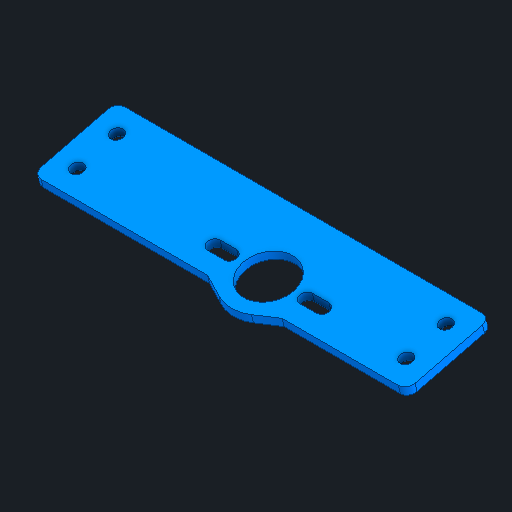
# Autodesk Inventor part: motor_mount_plate
Saved by Autodesk Inventor 2023 (Build 270158030, 158C)
## iProperties
Created: 2022-03-30
Part Number: motor_mount_plate
Material: Generic
Document SubType Name: Modeling
Designer: kardo
Density: 1 g/cm^3
Appearance: Blue Plastic
Author: kardo
Autodesk Inventor part; units mm, degrees
ref_plane "YZ Plane" through (0, 0, 0) normal (1, 0, 0) x (0, 1, 0)
ref_plane "XZ Plane" through (0, 0, 0) normal (0, 1, 0) x (-1, 0, 0)
ref_plane "XY Plane" through (0, 0, 0) normal (0, 0, 1) x (1, 0, 0)
derived "stencil_frame.ipt"
sketch "sk_cowl_joint_locations" plane through (54.6, 0, 0) normal (1, 0, 0) x (0, 1, 0)
  line L0 (-363, 18.496) -> (-275.8801, 20.463) construction
  arc A0 (-275.8801, 20.463) -> (-254.1001, 21.0191) centre (-359.1231, 3707.4463) ccw construction
  line L1 (-254.1001, 21.0191) -> (9.48, 28.5282) construction
  arc A1 (30.81, 28.832) -> (9.48, 28.5282) centre (30.81, -720.1791) ccw construction
  line L2 (30.81, 28.832) -> (94.8, 28.832) construction
  line L3 (94.8, 30.032) -> (30.81, 30.032) construction
  arc A2 (30.81, 30.032) -> (9.4458, 29.7277) centre (30.81, -720.1791) ccw construction
  line L4 (9.4458, 29.7277) -> (-254.1343, 22.2186) construction
  arc A3 (-275.9072, 21.6626) -> (-254.1343, 22.2186) centre (-359.1231, 3707.4463) ccw construction
  line L5 (-275.9072, 21.6626) -> (-363, 19.6963) construction
  line L6 (-242.0001, 4666.1952) -> (-242.0001, -2045.0469) construction
  line L7 (-120.9999, 4666.1952) -> (-120.9999, -2045.0469) construction
  line L8 (-363, 4666.1952) -> (-363, -2045.0469) construction
  line L9 (0, 4666.1952) -> (0, -2045.0469) construction
  line L10 (-242.0001, 45.0688) -> (-242.0001, 22.5643) construction
  line L11 (-120.9999, 49.9661) -> (-120.9999, 26.0115) construction
  line L12 (-363, 19.6963) -> (-363, 19.6963)
  line L13 (-363, 19.6963) -> (-363, 36.9211) construction
  line L14 (-1246.9714, 4491.7596) -> (383.4376, -2047.4538) construction
  line L15 (-362.7741, 36.9211) -> (-363, 39.712) construction
  line L16 (0, 51.6) -> (0, 29.4586) construction
  line L17 (-142.5135, 45.4866) -> (-137.5404, 25.5402) construction
  line L18 (-134.9025, 31.4945) -> (-138.7836, 30.5268) construction
  line L19 (-137.3891, 41.4677) -> (-141.2702, 40.5) construction
  line L20 (-142.5135, 45.4866) -> (-138.6324, 46.4543) construction
  line L21 (-137.5404, 25.5402) -> (-133.6592, 26.5079) construction
  line L22 (-138.6324, 46.4543) -> (-138.8117, 52.2515) construction
  spline S0 degree 2 poles (-363, 39.712) (-181.6483, 54.394) (0, 54.4) knots 0 0 0 1 1 1
  spline S1 degree 3 poles (0, 54.4) (31.284, 54.4) (68.256, 47.9917) (94.8, 37.536) knots 1 1 1 1 2 2 2 2
  spline S2 degree 3 poles (93.7738, 34.9308) (89.4268, 36.6431) (81.2968, 39.4556) (71.234, 42.2519) (63.4432, 44.1558) (58.1419, 45.3261) (51.4169, 46.6598) (45.9725, 47.6212) (39.1225, 48.6857) (33.6211, 49.4253) (26.7536, 50.2046) (21.2812, 50.7098) (14.5037, 51.1886) (7.8073, 51.5121) (2.5751, 51.6) (0, 51.6) knots 1 1 1 1 1.166667 1.291667 1.333333 1.416667 1.458333 1.541667 1.583333 1.666667 1.708333 1.791667 1.833333 1.916667 2 2 2 2
  spline S3 degree 3 poles (0, 51.6) (-20.1706, 51.5993) (-55.4643, 51.3605) (-95.7903, 50.6123) (-126.0307, 49.8474) (-146.1889, 49.2356) (-171.3841, 48.3435) (-191.5382, 47.528) (-216.7283, 46.3813) (-236.8783, 45.3621) (-262.0632, 43.9608) (-282.2091, 42.7379) (-307.3889, 41.082) (-332.5661, 39.2987) (-352.7052, 37.7363) (-362.7741, 36.9211) knots 0 0 0 0 0.166667 0.291667 0.333333 0.416667 0.458333 0.541667 0.583333 0.666666 0.708333 0.791666 0.833333 0.916666 1 1 1 1
  point P0 (0, 0)
  point P1 (-363, 28.3087)
  point P2 (-242.0001, 33.8165)
  point P3 (-120.9999, 37.9888)
  point P4 (0, 40.5293)
  point P5 (0, 40.5293)
ref_plane "plane_motor_mount" through (0, -127.05, 0) normal (0, 0.9702957, 0.2419219) x (-1, 0, 0)
ref_plane "plane_symmetry" through (0, 0, 0) normal (1, 0, 0) x (0, 1, 0)
sketch "sk_drivetrain_profile" plane through (6, 0, 0) normal (1, 0, 0) x (0, 1, 0)
  line L0 (-547.3485, 0) -> (393.091, 0) construction
  line L1 (-363, 4666.1952) -> (-363, -2045.0469) construction
  line L2 (0, 4666.1952) -> (0, -2045.0469) construction
  line L3 (-140.6277, 54.4571) -> (-133.8539, 27.2888)
  line L4 (-388, 0) -> (-343.0839, 2.7472)
  line L5 (-137.2408, 40.8729) -> (-226.9463, 18.5069)
  line L6 (-320.2745, 4.1423) -> (-272.9504, 7.0367) construction
  line L7 (-272.9504, 7.0367) -> (-226.9463, 18.5069) construction
  line L8 (-133.8539, 27.2888) -> (-133.8539, 22.2888) construction
  line L9 (-343.0839, 2.7472) -> (-320.2745, 4.1423)
  line L10 (-1246.9714, 4491.7596) -> (383.4376, -2047.4538) construction
  line L11 (-227.5223, 20.8174) -> (-137.8168, 43.1835) construction
  line L12 (-136.6647, 38.5624) -> (-226.3702, 16.1963) construction
  line L13 (-227.5223, 20.8174) -> (-226.3702, 16.1963) construction
  spline S0 degree 2 poles (-320.2745, 4.1423) (-272.9504, 7.0367) (-226.9463, 18.5069) knots 1 1 1 2 2 2
  line L14 (0, 21.4767) -> (-254.1001, 20.7404) construction
  line L15 (-55.6943, 22.5153) -> (-309.842, 21.7788) construction
  point P0 (0, 0)
  point P1 (-217.5636, 20.8462)
  point P2 (-207.6048, 20.8751)
  point P3 (-202.7352, 22.0892)
derived "parameters_frame.ipt"
sketch "sk_base" plane through (0, -127.05, 0) normal (0, 0.9702957, 0.2419219) x (-1, 0, 0)
  line L0 (0, -1635.5292) -> (0, 4543.1118) projected
  line L1 (-44.6, 47.8764) -> (-44.6, 27.3194)
  line L2 (-44.6, 27.3194) -> (0, 27.3194)
  line L3 (-44.6, 47.8764) -> (0, 47.8764)
  point P0 (0, -30.7362)
  point P1 (-54.6, 47.8764)
  point P2 (-54.6, 27.3194)
  dimension "d1" = 10
  constraints: 6 end point, 4 point on line, 2 perpendicular, 1 parallel
  measures "d1" distance from line of point (-54.6, 47.876) L1
extrude "base" add sketch "sk_base" against normal blind 2
sketch "sk_drill_joint" plane through (0, -127.05, 0) normal (0, 0.9702957, 0.2419219) x (-1, 0, 0)
  line L0 (-44.6, 47.8764) -> (-44.6, 27.3194) construction
  line L1 (-44.6, 47.8764) -> (0, 47.8764) construction
  line L2 (-44.6, 27.3194) -> (0, 27.3194) construction
  circle A0 centre (-39.2, 32.7194) radius 1.5
  circle A1 centre (-39.2, 42.4764) radius 1.5
  line L3 (-39.2, 42.4764) -> (-39.2, 47.8764) construction
  line L4 (-39.2, 42.4764) -> (-39.2, 32.7194) construction
  line L5 (-39.2, 32.7194) -> (-39.2, 27.3194) construction
  line L6 (-39.2, 42.4764) -> (-44.6, 42.4764) construction
  line L7 (-39.2, 32.7194) -> (-44.6, 32.7194) construction
  point P0 (0, -30.7362)
  dimension "d3" = 3
  dimension "d4" = 5.4
  constraints: 10 end point, 4 perpendicular, 4 point on line, 2 centre point, 2 collinear, 1 coincident, 1 equal radius, 1 parallel
  measures "d3" diameter of A1
  measures "d4" distance between parallel lines of L0 L4
extrude "drill_joint" cut sketch "sk_drill_joint" along normal through all both and the other way through all
mirror "mirror" about plane through (0, 0, 0) normal (1, 0, 0)
sketch "sk_expand_motor" plane through (0, -127.05, 0) normal (0, 0.9702957, 0.2419219) x (-1, 0, 0)
  line L0 (-6, 56.1242) -> (-6, 28.1242) construction
  line L1 (-9.8571, 50.2558) -> (-21.2857, 44.8347)
  arc A0 (-21.2857, 44.8347) -> (-21.2857, 39.4137) centre (-20, 42.1242) ccw
  line L2 (-21.2857, 39.4137) -> (-9.8571, 33.9926)
  arc A1 (-9.8571, 33.9926) -> (-2.1429, 33.9926) centre (-6, 42.1242) ccw
  line L3 (-2.1429, 33.9926) -> (9.2857, 39.4137)
  arc A2 (9.2857, 39.4137) -> (9.2857, 44.8347) centre (8, 42.1242) ccw
  line L4 (9.2857, 44.8347) -> (-2.1429, 50.2558)
  arc A3 (-2.1429, 50.2558) -> (-9.8571, 50.2558) centre (-6, 42.1242) ccw
  line L5 (-20, 42.1242) -> (8, 42.1242) construction
  point P0 (0, -30.7362)
  dimension "d23" = 28
  dimension "d24" = 18
  dimension "d26" = 6
  constraints: 10 end point, 8 point on circle, 8 tangent, 4 centre point, 3 midpoint, 2 coincident, 2 equal radius, 1 perpendicular
  measures "d23" distance of L5.end L5.start
  measures "d24" diameter of A3
  measures "d26" diameter of A2
extrude "expand_motor" add sketch "sk_expand_motor" against normal blind 2
sketch "sk_drill_motor" plane through (0, -127.05, 0) normal (0, 0.9702957, 0.2419219) x (-1, 0, 0)
  circle A0 centre (-6, 42.1242) radius 6
  line L0 (-15, 42.1242) -> (-19, 42.1242) construction
  line L1 (-15, 43.6242) -> (-19, 43.6242)
  line L2 (-19, 40.6242) -> (-15, 40.6242)
  arc A1 (-15, 40.6242) -> (-15, 43.6242) centre (-15, 42.1242) ccw
  arc A2 (-19, 43.6242) -> (-19, 40.6242) centre (-19, 42.1242) ccw
  line L3 (3, 42.1242) -> (7, 42.1242) construction
  line L4 (3, 40.6242) -> (7, 40.6242)
  line L5 (7, 43.6242) -> (3, 43.6242)
  arc A3 (3, 43.6242) -> (3, 40.6242) centre (3, 42.1242) ccw
  arc A4 (7, 40.6242) -> (7, 43.6242) centre (7, 42.1242) ccw
  line L6 (-15, 42.1242) -> (-6, 42.1242) construction
  line L7 (-6, 42.1242) -> (3, 42.1242) construction
  line L8 (-6, 56.1242) -> (-6, 28.1242) construction
  point P0 (0, -30.7362)
  point P1 (-17, 42.1242)
  point P2 (5, 42.1242)
  dimension "d9" = 12
  dimension "d14" = 3
  dimension "d15" = 4
  dimension "d21" = 18
  constraints: 20 end point, 8 point on circle, 8 tangent, 5 centre point, 5 collinear, 2 midpoint, 2 parallel, 1 equal radius, 1 perpendicular
  measures "d9" diameter of A0
  measures "d14" diameter of A2
  measures "d15" distance of L2.start L2.end
  measures "d21" distance of L3.start L0.start
extrude "drill_motor" cut sketch "sk_drill_motor" along normal through all both and the other way through all
fillet "round_corners" radius 2 4 edges at (44.6, -139.6026, 46.2123) (44.6, -134.6295, 26.266) (-44.6, -139.6026, 46.2123) (-44.6, -134.6295, 26.266)
derived "parameters_powertrain.ipt"
equation "\"d1\" = cowl_sealing_width + cowl_liner_width"
equation "\"d3\" = drill_motor_mount_diam"
equation "\"d4\" = 1.8 * drill_motor_mount_diam"
equation "\"d27\" = bulkhead_thickness"
equation "\"d18\" = 0.5 * bulkhead_inset"
equation "\"drill_motor_mount_diam\" = 3"
equation "\"bulkhead_thickness\" = 2"
equation "\"bulkhead_inset\" = 4"
equation "\"cowl_sealing_width\" = 5"
equation "\"cowl_liner_width\" = 5"
body "Solid1"
